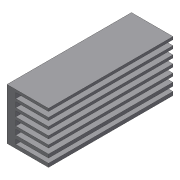
# Autodesk Inventor part: Jetson_Heatsink
Saved by Autodesk Inventor 2018 (Build 220112000, 112)
## iProperties
Created: 2019-09-10
Part Number: Jetson_Heatsink
Material: Generic
Document SubType Name: Modeling
Designer: Clevo
Density: 1 g/cm^3
Appearance: Default
Author: Clevo
Autodesk Inventor part; units mm, degrees
ref_plane "YZ Plane" through (0, 0, 0) normal (1, 0, 0) x (0, 1, 0)
ref_plane "XZ Plane" through (0, 0, 0) normal (0, 1, 0) x (-1, 0, 0)
ref_plane "XY Plane" through (0, 0, 0) normal (0, 0, 1) x (1, 0, 0)
sketch "Sketch1" plane through (0, 0, 0) normal (0, 1, 0) x (-1, 0, 0)
  line L0 (-10, -20) -> (10, -20)
  line L1 (10, -20) -> (10, 20)
  line L2 (10, 20) -> (-10, 20)
  line L3 (-10, 20) -> (-10, -20)
  line L4 (-10, -20) -> (10, 20) construction
  line L5 (10, -20) -> (-10, 20) construction
  point P0 (0, 0)
  dimension "d0" = 20
  dimension "d1" = 40
  constraints: 12 end point, 2 midpoint, 2 parallel, 1 horizontal, 1 perpendicular
  measures "d0" distance of L1.end L2.end
  measures "d1" distance of L0.end L1.end
extrude "Extrusion1" add sketch "Sketch1" along normal blind 60
sketch "Sketch2" plane through (0, 0, 0) normal (0, -1, 0) x (1, 0, 0)
  line L0 (10, -20) -> (-10, -20) projected
  line L1 (10, 20) -> (10, -20) projected
  line L2 (-10, 20) -> (10, 20) projected
  line L3 (-10, -20) -> (-10, 20) projected
  line L4 (10, 20) -> (10, -20) projected
  line L5 (10, 18.3) -> (-5.8, 18.3)
  line L6 (-5.8, 18.3) -> (-5.8, 16.1)
  line L7 (-5.8, 16.1) -> (10, 16.1)
  line L8 (10, 16.1) -> (10, 18.3)
  point P0 (0, 0)
  dimension "d4" = 1.7
  dimension "d5" = 4.2
  dimension "d6" = 2.2
  constraints: 8 end point, 2 parallel, 1 horizontal, 1 perpendicular, 1 point on line
  measures "d4" distance between parallel lines of L2 L5
  measures "d5" distance between parallel lines of L3 L6
  measures "d6" distance of L5.end L6.end
extrude "Extrusion2" cut sketch "Sketch2" against normal through all contours L7 L6 L5 L1
mirror "Mirror1" about plane through (0, 0, 0) normal (0, 0, 1) of "Extrusion2"
sketch "Sketch3" plane through (0, 0, 0) normal (0, -1, 0) x (1, 0, 0)
  line L0 (-5.8, -16.1) -> (10, -16.1) projected
  line L1 (10, 16.1) -> (10, -16.1) projected
  line L2 (10, 16.1) -> (-5.8, 16.1) projected
  line L3 (-5.8, 16.1) -> (-5.8, 18.3) projected
  line L4 (-5.8, 18.3) -> (10, 18.3) projected
  line L5 (10, 20) -> (10, 18.3) projected
  line L6 (-10, 20) -> (10, 20) projected
  line L7 (-10, -20) -> (-10, 20) projected
  line L8 (10, -20) -> (-10, -20) projected
  line L9 (10, -18.3) -> (10, -20) projected
  line L10 (10, -18.3) -> (-5.8, -18.3) projected
  line L11 (-5.8, -18.3) -> (-5.8, -16.1) projected
  line L12 (10, 14.8) -> (-5.8, 14.8)
  line L13 (-5.8, 14.8) -> (-5.8, 12.28)
  line L14 (-5.8, 12.28) -> (10, 12.28)
  line L15 (10, 12.28) -> (10, 14.8)
  point P0 (0, 0)
  dimension "d9" = 1.3
  dimension "d10" = 2.52
  constraints: 8 end point, 2 parallel, 1 collinear, 1 horizontal, 1 perpendicular, 1 point on line
  measures "d9" distance between parallel lines of L2 L12
  measures "d10" distance of L12.end L13.end
extrude "Extrusion3" cut sketch "Sketch3" against normal through all contours L14 L13 L12 L1
pattern_linear "Rectangular Pattern1" count 8 spacing 3.82 along (0, 0, -1) of "Extrusion3"
sketch "Sketch4" plane through (-10, 0, 20) normal (0, 0, 1) x (1, 0, 0)
  line L0 (-20.7139, 77.7692) -> (45.2661, 77.7692)
  line L1 (45.2661, 77.7692) -> (45.2661, -19.6204)
  line L2 (45.2661, -19.6204) -> (-20.7139, -19.6204)
  line L3 (-20.7139, -19.6204) -> (-20.7139, 77.7692)
  point P0 (10, 0)
  constraints: 8 end point, 2 parallel, 1 horizontal, 1 perpendicular
extrude "Extrusion4" cut sketch "Sketch4" against normal up to surface (15.36 mm away)
body "Solid1"
